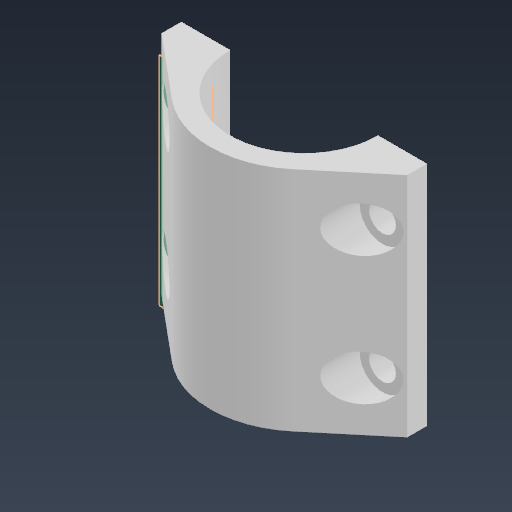
# Autodesk Inventor part: cpap hose holder
Saved by Autodesk Inventor 2024.3 (Build 283343000, 343)
## iProperties
Created: 2024-09-28
Part Number: cpap hose holder
Material: Generic
Document SubType Name: Modeling
Designer: MFil
Density: 1 g/cm^3
Appearance: Default
Author: MFil
Autodesk Inventor part; units mm, degrees
ref_plane "YZ Plane" through (0, 0, 0) normal (1, 0, 0) x (0, 1, 0)
ref_plane "XZ Plane" through (0, 0, 0) normal (0, 1, 0) x (-1, 0, 0)
ref_plane "XY Plane" through (0, 0, 0) normal (0, 0, 1) x (1, 0, 0)
sketch "Sketch1" plane through (0, 0, 0) normal (0, 1, 0) x (-1, 0, 0)
  arc A0 (-20.3357, 0) -> (-5.4696, 0) centre (-12.9027, 1) ccw projected
  circle A1 centre (-12.9027, 1) radius 7.5
  circle A2 centre (-12.9027, 1) radius 9.5
  line L0 (-0.4696, 0) -> (-5.4696, 0) projected
  line L1 (-20.3357, 0) -> (-25.3357, 0) projected
  line L2 (-0.4696, 0) -> (-25.3357, 0)
  line L3 (-25.3357, 0) -> (-25.3357, 1)
  line L4 (-25.3357, 1) -> (-0.4696, 1)
  line L5 (-0.4696, 1) -> (-0.4696, 0)
  line L6 (-0.4696, 1) -> (-25.3357, 1)
  line L7 (-25.3357, 1) -> (-25.3357, 3)
  line L8 (-25.3357, 3) -> (-0.4696, 3)
  line L9 (-0.4696, 3) -> (-0.4696, 1)
  line L10 (-25.3357, 3) -> (-16.9494, 9.9957)
  line L11 (-0.4696, 3) -> (-9.4027, 10.4518)
  point P0 (0, 0)
  point P1 (-6.8173, 8.2951)
  point P2 (-18.9881, 8.2951)
  point P3 (-20.4027, 1)
  point P4 (-5.4027, 1)
  dimension "d0" = 2
  dimension "d1" = 1
  dimension "d2" = 2
  constraints: 20 end point, 4 parallel, 2 horizontal, 2 perpendicular, 2 tangent, 1 centre point, 1 coincident, 3 other
  measures "d1" distance of L2.end L3.end
  measures "d2" distance of L6.end L7.end
ref_plane "Work Plane1" through (-1.0566, 20, -15.5001) normal (0, 1, 0) x (-0.6956029, 0, 0.7184265)
extrude "Extrusion1" add sketch "Sketch1" along normal blind 20 and the other way blind 3 contours L4 A2 L8 A1 | A1 L8 A2 L4 | L8 A2 A1 | L4 L7 L8 A2 | A2 L8 L9 L4 | L8 L10 A2 | A2 L11 L8
ref_plane "Work Plane2" through (5.4027, -3, 3) normal (0, 0, -1) x (-1, 0, 0)
sketch "Sketch2" plane through (5.4027, -3, 3) normal (0, 0, -1) x (-1, 0, 0)
  circle A0 centre (2.433, 5) radius 1.15 projected
  circle A1 centre (2.433, 18) radius 1.15 projected
  line L0 (-0.067, 23) -> (-0.067, 0) projected
  line L1 (4.933, 23) -> (-0.067, 23) projected
  line L2 (4.933, 23) -> (4.933, 0) projected
  line L3 (-0.067, 0) -> (4.933, 0) projected
  circle A2 centre (-17.433, 18) radius 1.15 projected
  circle A3 centre (-17.433, 5) radius 1.15 projected
  line L4 (-14.933, 0) -> (-14.933, 23) projected
  line L5 (-19.933, 0) -> (-14.933, 0) projected
  line L6 (-19.933, 23) -> (-19.933, 0) projected
  line L7 (-14.933, 23) -> (-19.933, 23) projected
  circle A4 centre (2.433, 18) radius 2.3
  circle A5 centre (2.433, 5) radius 2.3
  circle A6 centre (-17.433, 18) radius 2.3
  circle A7 centre (-17.433, 5) radius 2.3
  point P0 (5.4027, 3)
  dimension "d6" = 4.6
  dimension "d7" = 4.6
  dimension "d8" = 4.6
  dimension "d9" = 4.6
  constraints: 8 coincident, 4 centre point
  measures "d6" diameter of A4
  measures "d7" diameter of A5
  measures "d8" diameter of A6
  measures "d9" diameter of A7
extrude "Extrusion2" cut sketch "Sketch2" against normal blind 10 contours A0 | A1 | A2 | A3 | A4 | A5 | A6 | A7
hole "Hole1" at (2.9696, 15, 3) at (2.9696, 2, 3) at (22.8357, 2, 3) at (22.8357, 15, 3) direction (0, 0, -1) diameter 2.7 end through all clearance for "Countersunk Flat Head Screw ISO 2009/7046" size "M2.5" standard "ISO"
body "Solid1"
